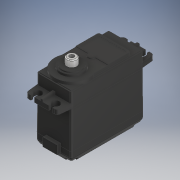
# Autodesk Inventor part: MG946R
Saved by Autodesk Inventor 2019.4 (Build 234330000, 330)
## iProperties
Created: 2018-10-02
Part Number: MG946R
Material: 一般
Document SubType Name: Modeling
Designer: TA
Density: 1 g/cm^3
Appearance: 滑らか - 黒
Author: TA
Autodesk Inventor part; units mm, degrees
sketch "スケッチ1" plane through (0, 0, 0) normal (0, 0, 1) x (1, 0, 0)
  line L0 (0, 0) -> (40.7, 0)
  line L1 (40.7, 0) -> (40.7, 19.7)
  line L2 (40.7, 19.7) -> (0, 19.7)
  line L3 (0, 19.7) -> (0, 0)
  dimension "d0" = 40.7
  dimension "d1" = 19.7
  constraints: 8 end point, 2 parallel, 1 horizontal, 1 perpendicular
  measures "d0" distance of L2.end L1.end
  measures "d1" distance of L1.end L0.end
extrude "押し出し1" add sketch "スケッチ1" along normal blind 6.5
sketch "スケッチ2" plane through (0, 0, 0) normal (0, 0, -1) x (-1, 0, 0)
  line L0 (0, 0) -> (-40.7, 0) projected
  line L1 (0, 19.7) -> (0, 0) projected
  line L2 (-40.7, 19.7) -> (0, 19.7) projected
  line L3 (-40.7, 0) -> (-40.7, 19.7) projected
ref_plane "作業平面1" through (0, 0, -20.5) normal (0, 0, -1) x (-1, 0, 0)
sketch "スケッチ3" plane through (0, 0, -20.5) normal (0, 0, -1) x (-1, 0, 0)
  line L0 (0, 0) -> (-40.7, 0) construction
  line L1 (0, 19.7) -> (0, 0) construction
  line L2 (-40.7, 19.7) -> (0, 19.7) construction
  line L3 (-40.7, 0) -> (-40.7, 19.7) construction
  line L4 (-40.55, 0.1) -> (-0.15, 0.1)
  line L5 (-0.15, 0.1) -> (-0.15, 19.6)
  line L6 (-0.15, 19.6) -> (-40.55, 19.6)
  line L7 (-40.55, 19.6) -> (-40.55, 0.1)
  line L8 (-40.7, 0) -> (-40.7, 19.7) projected
  line L9 (-40.7, 19.7) -> (0, 19.7) projected
  line L10 (-20.35, 19.7) -> (-20.35, 14.3498) construction
  line L11 (-40.7, 9.85) -> (-36.1597, 9.85) construction
  point P0 (-20.35, 19.6)
  point P1 (-40.55, 9.85)
  dimension "d5" = 40.4
  dimension "d6" = 19.5
  constraints: 12 end point, 4 midpoint, 2 horizontal, 2 parallel, 2 point on line, 1 perpendicular, 1 vertical
  measures "d5" distance of L6.end L5.end
  measures "d6" distance of L5.end L4.end
loft "ロフト1" add profiles "スケッチ3" section 1 edges at (20.35, 0, 0) (0, 9.85, 0) (20.35, 19.7, 0) (40.7, 9.85, 0)
sketch "スケッチ4" plane through (40.55, 0.1, -20.5) normal (0, 0, -1) x (-1, 0, 0)
  line L0 (0.075, 0.1) -> (40.325, 0.1)
  line L1 (40.325, 0.1) -> (40.325, 19.4)
  line L2 (40.325, 19.4) -> (0.075, 19.4)
  line L3 (0.075, 19.4) -> (0.075, 0.1)
  line L4 (40.4, 19.5) -> (0, 19.5) projected
  line L5 (-0.15, -0.1) -> (-0.15, 19.6) projected
  line L6 (20.2, 19.5) -> (20.2, 15.1197) construction
  line L7 (-0.15, 9.75) -> (1.9422, 9.75) construction
  point P0 (40.55, -0.1)
  point P1 (20.2, 19.4)
  point P2 (0.075, 9.75)
  dimension "d11" = 40.25
  dimension "d12" = 19.3
  constraints: 12 end point, 4 midpoint, 2 horizontal, 2 parallel, 2 point on line, 1 perpendicular, 1 vertical, 1 other
  measures "d11" distance of L2.end L1.end
  measures "d12" distance of L1.end L0.end
extrude "押し出し2" add sketch "スケッチ4" along normal blind 8.2
sketch "スケッチ5" plane through (40.475, 0.2, -20.5) normal (1, 0, 0) x (0, 0, -1)
  point P0 (-20.5, -0.2)
sketch "スケッチ6" plane through (0, 0, -20.5) normal (0, 0, -1) x (-1, 0, 0)
  line L0 (-40.475, 0.2) -> (-40.475, 19.5) construction
  line L1 (-40.475, 19.5) -> (-0.225, 19.5) construction
  line L2 (-0.225, 19.5) -> (-0.225, 0.2) construction
  line L3 (-0.225, 0.2) -> (-40.475, 0.2) construction
  line L4 (-40.55, 0.1) -> (-0.15, 0.1) construction
  line L5 (-0.15, 0.1) -> (-0.15, 19.6) construction
  line L6 (-0.15, 19.6) -> (-40.55, 19.6) construction
  line L7 (-40.55, 19.6) -> (-40.55, 0.1) construction
  line L8 (-0.225, 19.5) -> (-0.225, 0.2) projected
  line L9 (-0.225, 19.25) -> (6.65, 18.5)
  line L10 (6.65, 1.2) -> (-0.225, 0.45)
  line L11 (-0.225, 19.25) -> (-0.225, 0.45)
  line L12 (3.65, 20.854) -> (3.65, -5.0121) construction
  line L13 (3.65, 14.85) -> (4.0788, 18.7805) construction
  line L14 (3.65, 4.85) -> (4.0788, 0.9195) construction
  arc A0 (5.4966, 15.85) -> (5.4966, 13.85) centre (3.65, 14.85) ccw
  arc A1 (5.4966, 5.85) -> (5.4966, 3.85) centre (3.65, 4.85) ccw
  line L15 (5.4966, 15.85) -> (6.65, 15.85)
  line L16 (5.4966, 13.85) -> (6.65, 13.85)
  line L17 (5.4966, 5.85) -> (6.65, 5.85)
  line L18 (5.4966, 3.85) -> (6.65, 3.85)
  line L19 (6.65, 3.85) -> (6.65, 1.2)
  line L20 (6.65, 18.5) -> (6.65, 15.85)
  line L21 (6.65, 13.85) -> (6.65, 5.85)
  point P0 (0, 0)
  dimension "d15" = 18.8
  dimension "d16" = 19.3
  dimension "d17" = 0.25
  dimension "d19" = 17.3
  dimension "d21" = 10
  dimension "d22" = 4.2
  dimension "d23" = 4.2
  dimension "d24" = 2
  dimension "d25" = 1
  dimension "d26" = 2
  dimension "d27" = 1
  dimension "d28" = 6.875
  dimension "d98" = 3
  constraints: 26 end point, 14 perpendicular, 6 point on line, 4 point on circle, 3 collinear, 3 parallel, 2 centre point, 2 coincident, 2 equal length, 1 vertical
  measures "d15" distance of L10.end L9.start
  measures "d16" distance of L1.end L2.end
  measures "d17" distance of L10.end L2.end
  measures "d19" distance of L9.end L10.start
  measures "d21" distance of L13.start L14.start
  measures "d22" diameter of A0
  measures "d23" diameter of A1
  measures "d24" distance between parallel lines of L15 L16
  measures "d25" distance from line of L15 L13.start
  measures "d26" distance between parallel lines of L18 L17
  measures "d27" distance from line of L14.start L17
  measures "d28" distance between parallel lines of L11 L21
  measures "d98" distance between parallel lines of L21 L12
extrude "押し出し3" add sketch "スケッチ6" along normal blind 2.5
ref_plane "作業平面2" through (0.225, 9.85, -20.5) normal (0, -1, 0) x (1, 0, 0)
sketch "スケッチ7" plane through (0.225, 9.85, -20.5) normal (0, -1, 0) x (1, 0, 0)
  line L0 (-6.875, 0) -> (-0.075, 0) projected
  line L1 (-6.875, 0) -> (-6.875, -2.5) projected
  line L2 (0, -2.5) -> (-6.875, -2.5) projected
  line L3 (0, 0) -> (0, -2.5) projected
  line L4 (-0.075, 0) -> (0, 0) projected
  line L5 (0, 0) -> (40.25, 0) projected
  line L6 (0, 0) -> (0, -8.2) projected
  line L7 (40.25, -8.2) -> (0, -8.2) projected
  line L8 (40.25, 0) -> (40.25, -8.2) projected
  line L9 (-6.875, -2.5) -> (-6.875, -3.7)
  line L10 (-6.875, -3.7) -> (0, -4.2)
  line L11 (0, -4.2) -> (0, -2.5)
  line L12 (-6.875, -2.5) -> (0, -2.5)
  point P0 (-0.225, 20.5)
  dimension "d31" = 1.2
  dimension "d32" = 1.7
  constraints: 8 end point, 1 collinear, 1 horizontal, 1 point on line, 1 vertical
  measures "d31" distance of L1.end L9.end
  measures "d32" distance of L2.start L10.end
extrude "押し出し4" add sketch "スケッチ7" along normal mid plane 1.3 contours L2 L6 L10 L9
ref_plane "作業平面3" through (20.35, 0.2, -28.7) normal (-1, 0, 0) x (0, 0, 1)
mirror "ミラー1" about plane through (20.35, 0.2, -28.7) normal (-1, 0, 0) of "押し出し4", "押し出し3"
fillet "フィレット2" radius 1.5 4 edges at (47.35, 1.2, -21.75) (47.35, 18.5, -21.75) (-6.65, 1.2, -21.75) (-6.65, 18.5, -21.75)
chamfer "面取り1" distance 1.5 distance2 3 1 edges at (20.35, 0, 6.5) measured on face at (20.35, 0.5, 6.5)
chamfer "面取り2" distance 1.5 distance2 3 1 edges at (20.35, 19.7, 6.5) measured on face at (20.35, 19.2, 6.5)
chamfer "面取り3" distance 1.5 distance2 3 1 edges at (40.7, 9.85, 6.5) measured on face at (40.2, 9.85, 6.5)
chamfer "面取り4" distance 1.5 distance2 3 1 edges at (0, 9.85, 6.5) measured on face at (0.5, 9.85, 6.5)
sketch "スケッチ8" plane through (0, 0, 6.5) normal (0, 0, 1) x (1, 0, 0)
  line L0 (0, 19.7) -> (0, 0) construction
  line L1 (0, 0) -> (40.7, 0) construction
  line L2 (40.7, 19.7) -> (0, 19.7) construction
  line L3 (40.7, 0) -> (40.7, 19.7) construction
  line L4 (1.5, 1.5) -> (1.5, 18.2) construction
  line L5 (39.2, 1.5) -> (1.5, 1.5) construction
  line L6 (39.2, 18.2) -> (39.2, 1.5) construction
  line L7 (1.5, 18.2) -> (39.2, 18.2) construction
  arc A0 (4.55, 2.35) -> (2.55, 4.35) centre (2.55, 2.35) ccw
  line L8 (4.55, 2.35) -> (4.55, 0)
  line L9 (2.55, 4.35) -> (0, 4.35)
  line L10 (0, 19.7) -> (0, 0) projected
  line L11 (0, 4.35) -> (0, 0)
  line L12 (0, 0) -> (4.55, 0)
  dimension "d49" = 2.55
  dimension "d50" = 2.35
  dimension "d51" = 4
  constraints: 8 end point, 4 perpendicular, 2 point on circle, 2 point on line, 2 tangent, 1 centre point, 1 coincident
  measures "d49" distance from line of L0 point (2.55, 2.35)
  measures "d50" distance from line of L1 point (2.55, 2.35)
  measures "d51" diameter of A0
extrude "押し出し5" cut sketch "スケッチ8" against normal blind 1.4
sketch "スケッチ9" plane through (0, 0, 5.1) normal (0, 0, 1) x (1, 0, 0)
  arc A0 (4.55, 2.35) -> (2.55, 4.35) centre (2.55, 2.35) ccw construction
  point P0 (0, 0)
hole "穴1" at (2.55, 2.35, 5.1) direction (0, 0, -1) diameter 2 depth 30 tip angle 118
mirror "ミラー2" about plane through (0.225, 9.85, -20.5) normal (0, -1, 0) of "押し出し5", "穴1"
mirror "ミラー3" about plane through (20.35, 0.2, -28.7) normal (-1, 0, 0) of "押し出し5", "穴1", "ミラー2"
fillet "フィレット3" radius 1 16 edges at (0.075, 19.65, -10.25) (0.225, 19.5, -24.6) (0, 19.7, 1.75) (0.4, 19.3, 4.3) (0.225, 0.2, -24.6) (0.075, 0.05, -10.25) (0, 0, 1.75) (40.475, 0.2, -24.6) (40.625, 0.05, -10.25) (40.7, 0, 1.75) (40.475, 19.5, -24.6) (40.625, 19.65, -10.25) (40.3, 19.3, 4.3) (40.7, 19.7, 1.75) (0.4, 0.4, 4.3) (40.3, 0.4, 4.3)
fillet "フィレット4" radius 2 16 edges at (39.7503, 0.0013, 3.5025) (40.4071, 0.2929, 3.5818) (40.6987, 0.9497, 3.5025) (40.7, 9.85, 3.5) (40.6987, 18.7503, 3.5025) (40.4071, 19.4071, 3.5818) (39.7503, 19.6987, 3.5025) (20.35, 19.7, 3.5) (0.9497, 19.6987, 3.5025) (0.2929, 19.4071, 3.5818) (0.0013, 18.7503, 3.5025) (0, 9.85, 3.5) (0.0013, 0.9497, 3.5025) (0.2929, 0.2929, 3.5818) (0.9497, 0.0013, 3.5025) (20.35, 0, 3.5)
sketch "スケッチ10" plane through (40.55, 0.1, -28.7) normal (0, 0, -1) x (-1, 0, 0)
  arc A0 (1.075, 19.4) -> (0.075, 18.4) centre (1.075, 18.4) ccw construction
  line L0 (0.075, 18.4) -> (0.075, 1.1) construction
  arc A1 (0.075, 1.1) -> (1.075, 0.1) centre (1.075, 1.1) ccw construction
  line L1 (1.075, 0.1) -> (39.325, 0.1) construction
  arc A2 (39.325, 0.1) -> (40.325, 1.1) centre (39.325, 1.1) ccw construction
  line L2 (40.325, 1.1) -> (40.325, 18.4) construction
  arc A3 (40.325, 18.4) -> (39.325, 19.4) centre (39.325, 18.4) ccw construction
  line L3 (39.325, 19.4) -> (1.075, 19.4) construction
  line L4 (39.325, 0.6) -> (1.075, 0.6)
  arc A4 (0.575, 1.1) -> (1.075, 0.6) centre (1.075, 1.1) ccw
  line L5 (0.575, 1.1) -> (0.575, 18.4)
  arc A5 (1.075, 18.9) -> (0.575, 18.4) centre (1.075, 18.4) ccw
  line L6 (1.075, 18.9) -> (39.325, 18.9)
  arc A6 (39.825, 18.4) -> (39.325, 18.9) centre (39.325, 18.4) ccw
  line L7 (39.825, 18.4) -> (39.825, 1.1)
  arc A7 (39.325, 0.6) -> (39.825, 1.1) centre (39.325, 1.1) ccw
  point P0 (40.55, -0.1)
  dimension "d63" = 0.5
  constraints: 8 end point, 8 point on circle, 4 centre point, 7 other
  measures "d63" distance between parallel lines of L1 L4
extrude "押し出し6" add sketch "スケッチ10" along normal blind 0.5
sketch "スケッチ11" plane through (40.55, 0.1, -29.2) normal (0, 0, -1) x (-1, 0, 0)
  line L0 (53.2603, 9.75) -> (-20.2506, 9.75) construction
  line L1 (39.325, 18.9) -> (1.075, 18.9) construction
  line L2 (1.075, 0.6) -> (39.325, 0.6) construction
  arc A0 (26.9323, 0.825) -> (26.9323, 18.675) centre (30.4, 9.75) ccw
  line L3 (26.9323, 0.825) -> (6.375, 0.825)
  line L4 (6.375, 0.825) -> (6.375, 18.675)
  line L5 (6.375, 18.675) -> (26.9323, 18.675)
  line L6 (40.325, 1.1) -> (40.325, 18.4) projected
  line L7 (0.075, 18.4) -> (0.075, 1.1) projected
  point P0 (40.55, -0.1)
  point P1 (6.375, 9.75)
  dimension "d66" = 18.3
  dimension "d67" = 9.15
  dimension "d68" = 19.15
  dimension "d69" = 17.85
  dimension "d70" = 24.025
  dimension "d73" = 6.3
  constraints: 8 end point, 2 horizontal, 2 point on circle, 2 point on line, 1 centre point, 1 midpoint, 1 parallel, 1 perpendicular
  measures "d66" distance between parallel lines of L1 L2
  measures "d67" distance between parallel lines of L2 L0
  measures "d68" diameter of A0
  measures "d69" distance of L3.end L4.end
  measures "d70" distance from line of A0.centre L4
  measures "d73" distance between parallel lines of L7 L4
extrude "押し出し7" add sketch "スケッチ11" against normal blind 0.5 and the other way blind 1.65
fillet "フィレット5" radius 1 2 edges at (34.175, 18.775, -30.025) (34.175, 0.925, -30.025)
sketch "スケッチ12" plane through (40.55, 0.1, -30.85) normal (0, 0, -1) x (-1, 0, 0)
  arc A0 (6.375, 1.825) -> (7.375, 0.825) centre (7.375, 1.825) ccw construction
  line L0 (7.375, 0.825) -> (26.9323, 0.825) construction
  arc A1 (26.9323, 0.825) -> (26.9323, 18.675) centre (30.4, 9.75) ccw construction
  line L1 (26.9323, 18.675) -> (7.375, 18.675) construction
  arc A2 (7.375, 18.675) -> (6.375, 17.675) centre (7.375, 17.675) ccw construction
  line L2 (6.375, 17.675) -> (6.375, 1.825) construction
  circle A3 centre (30.4, 9.75) radius 6.425
  point P0 (40.55, -0.1)
  dimension "d79" = 12.85
  constraints: 1 centre point, 1 coincident
  measures "d79" diameter of A3
extrude "押し出し8" add sketch "スケッチ12" along normal blind 1.3
sketch "スケッチ14" plane through (10.15, 9.85, -32.15) normal (0, 0, -1) x (-1, 0, 0)
  circle A0 centre (0, 0) radius 5.55
  circle A1 centre (0, 0) radius 6.425 construction
  point P0 (10.15, -9.85)
  dimension "d82" = 11.1
  constraints: 1 centre point, 1 coincident
  measures "d82" diameter of A0
extrude "押し出し9" add sketch "スケッチ14" along normal blind 0.7
sketch "スケッチ15" plane through (10.15, 9.85, -32.85) normal (0, 0, -1) x (-1, 0, 0)
  circle A0 centre (0, 0) radius 2.75
  point P0 (10.15, -9.85)
  dimension "d85" = 5.5
  constraints: 1 centre point, 1 coincident
  measures "d85" diameter of A0
extrude "押し出し10" add sketch "スケッチ15" along normal blind 3.65 separate body
sketch "スケッチ16" plane through (10.15, 9.85, -36.5) normal (0, 0, -1) x (-1, 0, 0)
  point P0 (10.15, -9.85)
  point P1 (0, 0)
hole "穴2" at (10.15, 9.85, -36.5) direction (0, 0, 1) diameter 2.459 depth 5.5 bodies 2 thread size "M3x0.5" class "6H" standard "ISO Metric profile"
chamfer "面取り5" distance 0.5 angle 45 1 edges at (12.9, 9.85, -36.5)
sketch "スケッチ18" plane through (40.55, 0.1, -30.85) normal (0, 0, -1) x (-1, 0, 0)
  circle A0 centre (30.4, 9.75) radius 6.425 projected
  arc A1 (6.375, 1.825) -> (7.375, 0.825) centre (7.375, 1.825) ccw projected
  line L0 (7.375, 0.825) -> (26.9323, 0.825) projected
  arc A2 (26.9323, 0.825) -> (26.9323, 18.675) centre (30.4, 9.75) ccw projected
  line L1 (26.9323, 18.675) -> (7.375, 18.675) projected
  arc A3 (7.375, 18.675) -> (6.375, 17.675) centre (7.375, 17.675) ccw projected
  line L2 (6.375, 17.675) -> (6.375, 1.825) projected
  line L3 (26.9323, 0.825) -> (7.375, 0.825) projected
  line L4 (19.175, 0.825) -> (19.175, 18.675)
  line L5 (26.9323, 18.675) -> (7.375, 18.675) projected
  point P0 (40.55, -0.1)
  dimension "d99" = 12.8
  constraints: 2 end point, 2 point on line, 1 perpendicular
  measures "d99" distance between parallel lines of L2 L4
extrude "押し出し11" add sketch "スケッチ18" along normal blind 0.4 contours L2 A3 L1 L4 L0 A1 bodies 1
sketch "スケッチ19" plane through (40.55, 0.1, -30.85) normal (0, 0, -1) x (-1, 0, 0)
  line L0 (19.175, 18.675) -> (19.175, 0.825) construction
  line L1 (19.175, 0.825) -> (26.9323, 0.825) construction
  arc A0 (26.9323, 0.825) -> (26.9323, 18.675) centre (30.4, 9.75) ccw construction
  line L2 (26.9323, 18.675) -> (19.175, 18.675) construction
  circle A1 centre (30.4, 9.75) radius 6.425 construction
  line L3 (19.175, 0.825) -> (19.175, 18.675) construction
  line L4 (19.175, 18.675) -> (7.375, 18.675) construction
  arc A2 (7.375, 18.675) -> (6.375, 17.675) centre (7.375, 17.675) ccw construction
  line L5 (6.375, 17.675) -> (6.375, 1.825) construction
  arc A3 (6.375, 1.825) -> (7.375, 0.825) centre (7.375, 1.825) ccw construction
  line L6 (7.375, 0.825) -> (19.175, 0.825) construction
  line L7 (19.175, 0.825) -> (19.175, 18.675) construction
  circle A4 centre (19.175, 9.75) radius 2.05
  line L8 (19.175, 18.675) -> (19.175, 0.825) construction
  point P0 (40.55, -0.1)
  dimension "d102" = 4.1
  dimension "d103" = 17.85
  dimension "d104" = 8.925
  constraints: 1 centre point, 1 midpoint
  measures "d102" diameter of A4
  measures "d103" distance of L0.start L0.end
  measures "d104" distance of L0.end A4.centre
extrude "押し出し12" add sketch "スケッチ19" along normal blind 0.5 bodies 1
sketch "スケッチ20" plane through (21.375, 9.85, -31.35) normal (0, 0, -1) x (-1, 0, 0)
  arc A0 (0, 2.05) -> (0, -2.05) centre (0, 0) ccw projected
  line L0 (0, 2.05) -> (0, 8.925) projected
  line L1 (0, 8.925) -> (-11.8, 8.925) projected
  arc A1 (-11.8, 8.925) -> (-12.8, 7.925) centre (-11.8, 7.925) ccw projected
  line L2 (-12.8, 7.925) -> (-12.8, -7.925) projected
  arc A2 (-12.8, -7.925) -> (-11.8, -8.925) centre (-11.8, -7.925) ccw projected
  line L3 (-11.8, -8.925) -> (0, -8.925) projected
  line L4 (0, -8.925) -> (0, -2.05) projected
  line L5 (-1.3, 7.625) -> (-1.3, 1.5851)
  line L6 (-1.3, 1.5851) -> (-1.3, -7.625)
  line L7 (-1.3, -7.625) -> (-11.5, -7.625)
  line L8 (-11.5, -7.625) -> (-11.5, 7.625)
  line L9 (-11.5, 7.625) -> (-1.3, 7.625)
  point P0 (21.375, -9.85)
  dimension "d108" = 1.3
  constraints: 10 end point, 1 collinear, 1 point on circle, 2 other
  measures "d108" distance between parallel lines of L0 L5
extrude "押し出し13" cut sketch "スケッチ20" against normal blind 0.3 contours L6 A0 | A0 L6 L7 L8 L9 L5 bodies 1
ref_plane "作業平面5" through (1.225, 9.85, -20.5) normal (0, 1, 0) x (1, 0, 0)
sketch "スケッチ21" plane through (0, 1, 0) normal (-1, 0, 0) x (0, 0, 1)
  line L0 (3.2, 4.85) -> (-1.5, 4.85)
  line L1 (-1.5, 4.85) -> (-1.5, 12.85)
  line L2 (-1.5, 12.85) -> (3.2, 12.85)
  line L3 (3.0279, 17.7) -> (3.0279, 0) projected
  line L4 (0, 17.7) -> (3.0279, 17.7) projected
  line L5 (0, 17.7) -> (0, 0) projected
  line L6 (3.0279, 0) -> (0, 0) projected
  line L7 (3.2, 4.85) -> (3.2, 12.85)
  line L8 (6.5, 3.35) -> (6.5, 14.35) projected
  point P0 (0, -1)
  dimension "d111" = 8
  dimension "d112" = 4.7
  dimension "d113" = 17.7
  dimension "d114" = 4.85
  dimension "d122" = 3.3
  constraints: 8 end point, 1 horizontal, 1 parallel, 1 perpendicular, 1 vertical
  measures "d111" distance of L0.end L1.end
  measures "d112" distance of L0.start L0.end
  measures "d113" distance of L4.start L5.end
  measures "d114" distance between parallel lines of L4 L2
  measures "d122" distance between parallel lines of L8 L7
extrude "押し出し14" add sketch "スケッチ21" along normal blind 2 and the other way blind 1 contours L0 L3 L2 L7 | L0 L5 L2 L3 | L0 L1 L2 L5 bodies 1
ref_plane "作業平面4" through (20.35, 0.2, -28.7) normal (-1, 0, 0) x (0, 0, 1)
equation "\"d17\" = -0.5 * d15 + 0.5 * d16"
equation "\"d23\" = d22"
equation "\"d26\" = d24"
equation "\"d67\" = 0.5 * d66"
equation "\"d104\" = 0.5 * d103"
equation "\"d114\" = -0.5 * d111 + 0.5 * d113"
